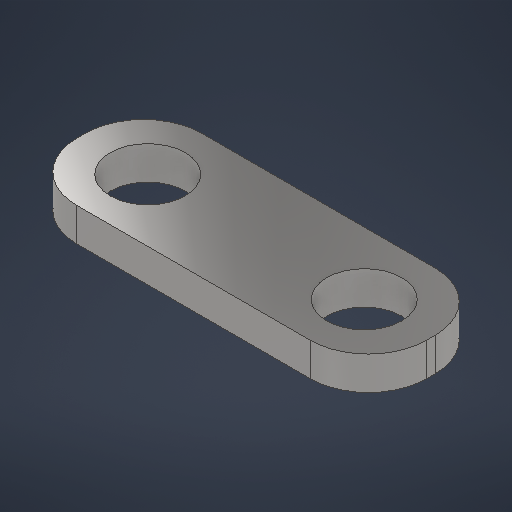
# Autodesk Inventor part: Plate
Saved by Autodesk Inventor 2026 (Build 300175050, 175E)
## iProperties
Created: 2026-02-19
Part Number: Plate
Material: 鋼、軟鋼
Document SubType Name: Modeling
Designer: hirotaka-honda
Density: 7.85 g/cm^3
Appearance: 半つや出し
Author: hirotaka-honda
Autodesk Inventor part; units mm, degrees
ref_plane "YZ Plane" through (0, 0, 0) normal (1, 0, 0) x (0, 1, 0)
ref_plane "XZ Plane" through (0, 0, 0) normal (0, 1, 0) x (-1, 0, 0)
ref_plane "XY Plane" through (0, 0, 0) normal (0, 0, 1) x (1, 0, 0)
sketch "スケッチ1" plane through (0, 0, 0) normal (0, 1, 0) x (-1, 0, 0)
  line L0 (0, 0) -> (-21, 0)
  line L1 (-21, 0) -> (-21, -7.5)
  line L2 (-21, -7.5) -> (0, -7.5)
  line L3 (0, -7.5) -> (0, 0)
  dimension "d1" = 21
  dimension "d27" = 7.5
  constraints: 8 end point, 2 parallel, 1 horizontal, 1 perpendicular
  measures "d1" distance of L1.end L2.end
  measures "d27" distance between parallel lines of L0 L2
extrude "押し出し1" add sketch "スケッチ1" along normal blind 2
sketch "スケッチ2" plane through (0, 2, 0) normal (0, 1, 0) x (1, 0, 0)
  line L0 (0, 7.5) -> (0, 0) projected
  line L1 (0, 3.75) -> (21, 3.75)
  line L2 (21, 0) -> (21, 7.5) projected
  line L3 (0, 0) -> (21, 0) projected
  line L4 (10.5, 0) -> (10.5, 7.5)
  line L5 (21, 7.5) -> (0, 7.5) projected
  line L6 (4, 0) -> (4, 7.5)
  line L7 (17, 0) -> (17, 7.5)
  point P0 (4, 3.75)
  point P1 (17, 3.75)
  dimension "d18" = 3.75
  dimension "d19" = 3.75
  dimension "d20" = 21
  dimension "d23" = 4
  dimension "d24" = 4
  constraints: 8 end point, 6 midpoint, 4 point on line, 2 parallel
  measures "d18" distance between parallel lines of L1 L3
  measures "d19" distance between parallel lines of L1 L5
  measures "d20" distance between parallel lines of L2 L0
  measures "d23" distance between parallel lines of L0 L6
  measures "d24" distance between parallel lines of L2 L7
hole "穴1" at (4, 2, -3.75) at (17, 2, -3.75) direction (0, -1, 0) diameter 4.5 end through all
fillet "フィレット1" radius 3.5 4 edges at (21, 1, 0) (21, 1, -7.5) (0, 1, 0) (0, 1, -7.5)
